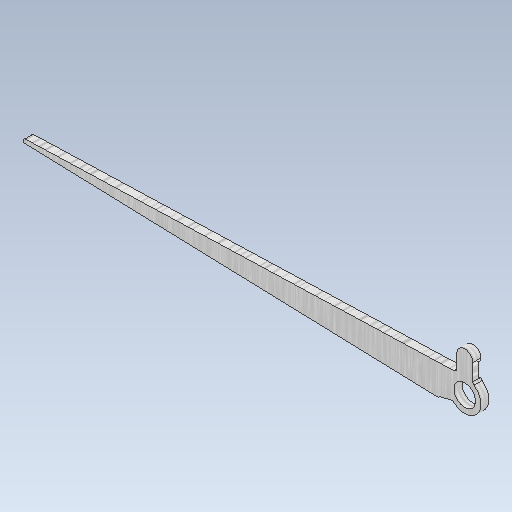
# Autodesk Inventor part: アーム先端
Saved by Autodesk Inventor 2020.2 (Build 242310000, 310)
## iProperties
Created: 2020-03-28
Part Number: アーム先端
Material: アルミニウム 7075
Document SubType Name: Modeling
Designer: aoyam
Density: 2.81 g/cm^3
Appearance: サテン - ブラシ仕上げ 重厚
Mass: 8.77948 g
Surface Area: 37.1512 cm^2
Volume: 3.12437 cm^3
Author: aoyam
Autodesk Inventor part; units mm, degrees
ref_plane "YZ Plane" through (0, 0, 0) normal (1, 0, 0) x (0, 1, 0)
ref_plane "XZ Plane" through (0, 0, 0) normal (0, 1, 0) x (-1, 0, 0)
ref_plane "XY Plane" through (0, 0, 0) normal (0, 0, 1) x (1, 0, 0)
sketch "スケッチ1" plane through (0, 0, 0) normal (0, 0, 1) x (1, 0, 0)
  line L0 (0, 0) -> (-164, 0)
  circle A0 centre (0, 0) radius 4.025
  line L1 (0, 0) -> (0, 12)
  circle A1 centre (0, 0) radius 6
  line L2 (0, 0) -> (0, 12) construction
  line L3 (3, 0) -> (3, 12)
  line L4 (-3, 12) -> (-3, 0)
  arc A2 (-3, 0) -> (3, 0) centre (0, 0) ccw
  arc A3 (3, 12) -> (-3, 12) centre (0, 12) ccw
  circle A4 centre (-164, 0) radius 0.75
  line L5 (-164.024, 0.7496) -> (-0.1921, 5.9969)
  line L6 (-0.1921, -5.9969) -> (-164.024, -0.7496)
  line L7 (-4.4505, -4.0241) -> (-11.6988, -5.6284)
  circle A5 centre (-7.8489, -7.8489) radius 3
  line L8 (0, 0) -> (-7.8489, -7.8489)
  line L9 (-139.5205, 0) -> (-135.0205, 7.7942)
  line L10 (-135.0205, 7.7942) -> (-164.1766, 0.7289)
  point P0 (0, 6)
  point P1 (3, 5.1962)
  point P2 (-3, 5.1962)
  point P3 (-8.4972, -4.9198)
  point P4 (-4.2426, -4.2426)
  point P5 (-9.9269, -5.6851)
  point P6 (-3, 5.907)
  point P7 (-138.6179, 1.5633)
  dimension "d2" = 164
  dimension "d3" = 8.05
  dimension "d4" = 12
  dimension "d5" = 90
  dimension "d7" = 6
  dimension "d8" = 1.5
  dimension "d13" = 6
  dimension "d14" = 45
  dimension "d21" = 12
  dimension "d23" = 11.1
  dimension "d33" = 30
  dimension "d34" = 9
  dimension "d35" = 60
  constraints: 24 end point, 10 point on circle, 10 tangent, 6 centre point, 2 coincident, 2 point on line, 1 horizontal, 1 midpoint, 1 parallel
  measures "d2" distance of L0.start L0.end
  measures "d3" diameter of A0
  measures "d4" distance of L1.start L1.end
  measures "d5" angle of L1 L0
  measures "d7" diameter of A3
  measures "d8" diameter of A4
  measures "d13" diameter of A5
  measures "d14" angle of L8 L0
  measures "d21" diameter of A1
  measures "d23" distance of L8.end L0.start
  measures "d33" distance of L9.end L10.end
  measures "d34" distance of L9.start L9.end
  measures "d35" angle of L0 L9
extrude "押し出し1" add sketch "スケッチ1" along normal blind 3 contours L1 A1 L3 A0 | A0 L4 A1 L1 | A0 L8 A1 L0 | L0 A1 L4 A0 | L3 A1 L8 A0 | A1 L5 L4 A3 L3 | A1 L7 L6 A4 L0 | L0 L9 L5 L4 A1 | L4 L5 A1 | L0 A4 L5 L9 | A4 | A5 L6 L7
fillet "フィレット1" radius 1.05 2 edges at (3, 5.1962, 1.5) (-9.9269, -5.6851, 1.5)
sketch "スケッチ2" plane through (0, 0, 3) normal (0, 0, 1) x (1, 0, 0)
  arc A0 (-10.3309, -5.6722) -> (-9.6625, -5.4591) centre (-10.2972, -4.6227) ccw projected
  arc A1 (-8.4972, -4.9198) -> (-9.6625, -5.4591) centre (-7.8489, -7.8489) ccw projected
  arc A2 (-4.4505, -4.0241) -> (3.4468, 4.9112) centre (0, 0) ccw projected
  arc A3 (3, 5.7706) -> (3.4468, 4.9112) centre (4.05, 5.7706) ccw projected
  line L0 (3, 5.7706) -> (3, 12) projected
  arc A4 (3, 12) -> (-3, 12) centre (0, 12) ccw projected
  line L1 (-3, 12) -> (-3, 5.907) projected
  line L2 (-3, 5.907) -> (-164.024, 0.7496) projected
  arc A5 (-164.024, 0.7496) -> (-164.024, -0.7496) centre (-164, 0) ccw projected
  line L3 (-164.024, -0.7496) -> (-10.3309, -5.6722) projected
  circle A6 centre (0, 0) radius 4.025 projected
  line L4 (-8.4972, -4.9198) -> (-4.4505, -4.0241) projected
fillet "フィレット3" radius 1.05 2 edges at (-4.4505, -4.0241, 1.5) (-3, 5.907, 1.5)
sketch "スケッチ4" plane through (0, 0, 0) normal (0, 0, -1) x (-1, 0, 0)
  circle A0 centre (0, 0) radius 4.025 projected
  arc A1 (9.6625, -5.4591) -> (10.3309, -5.6722) centre (10.2972, -4.6227) ccw projected
  line L0 (164.024, -0.7496) -> (10.3309, -5.6722) projected
  arc A2 (164.024, -0.7496) -> (164.024, 0.7496) centre (164, 0) ccw projected
  line L1 (4.0164, 5.8744) -> (164.024, 0.7496) projected
  arc A3 (3, 6.9239) -> (4.0164, 5.8744) centre (4.05, 6.9239) ccw projected
  line L2 (3, 12) -> (3, 6.9239) projected
  arc A4 (3, 12) -> (-3, 12) centre (0, 12) ccw projected
  line L3 (-3, 5.7706) -> (-3, 12) projected
  arc A5 (-3.4468, 4.9112) -> (-3, 5.7706) centre (-4.05, 5.7706) ccw projected
  arc A6 (-3.4468, 4.9112) -> (4.0752, -4.4037) centre (0, 0) ccw projected
  arc A7 (5.0153, -4.1491) -> (4.0752, -4.4037) centre (4.7884, -5.1743) ccw projected
  line L4 (8.4972, -4.9198) -> (5.0153, -4.1491) projected
  arc A8 (9.6625, -5.4591) -> (8.4972, -4.9198) centre (7.8489, -7.8489) ccw projected
  circle A9 centre (15.0911, 0) radius 2
  circle A10 centre (80.8845, 0) radius 1.05
  line L5 (15.12, 1.9998) -> (80.8997, 1.0499)
  line L6 (80.8997, -1.0499) -> (15.12, -1.9998)
  line L7 (0, 0) -> (80.8845, 0)
  dimension "d24" = 4
  dimension "d25" = 2.1
  constraints: 6 end point, 4 point on circle, 4 tangent, 2 centre point, 1 horizontal, 1 point on line
  measures "d24" diameter of A9
  measures "d25" diameter of A10
extrude "押し出し3" cut sketch "スケッチ4" against normal blind 1.5 contours L7 A9 | L7 A10 L6 A9 | A9 L7 | A9 L5 A10 L7 | A10
sketch "スケッチ5" plane through (0, 0, 0) normal (0, 0, -1) x (-1, 0, 0)
  line L0 (80.8997, -1.0499) -> (15.12, -1.9998) projected
  arc A0 (15.12, 1.9998) -> (15.12, -1.9998) centre (15.0911, 0) ccw projected
  line L1 (15.12, 1.9998) -> (80.8997, 1.0499) projected
  arc A1 (80.8997, -1.0499) -> (80.8997, 1.0499) centre (80.8845, 0) ccw projected
  circle A2 centre (0, 0) radius 4.025 projected
  arc A3 (9.6625, -5.4591) -> (10.3309, -5.6722) centre (10.2972, -4.6227) ccw projected
  line L2 (164.024, -0.7496) -> (10.3309, -5.6722) projected
  arc A4 (164.024, -0.7496) -> (164.024, 0.7496) centre (164, 0) ccw projected
  line L3 (4.0164, 5.8744) -> (164.024, 0.7496) projected
  arc A5 (3, 6.9239) -> (4.0164, 5.8744) centre (4.05, 6.9239) ccw projected
  line L4 (3, 12) -> (3, 6.9239) projected
  arc A6 (3, 12) -> (-3, 12) centre (0, 12) ccw projected
  line L5 (-3, 5.7706) -> (-3, 12) projected
  arc A7 (-3.4468, 4.9112) -> (-3, 5.7706) centre (-4.05, 5.7706) ccw projected
  arc A8 (-3.4468, 4.9112) -> (4.0752, -4.4037) centre (0, 0) ccw projected
  arc A9 (5.0153, -4.1491) -> (4.0752, -4.4037) centre (4.7884, -5.1743) ccw projected
  line L6 (8.4972, -4.9198) -> (5.0153, -4.1491) projected
  arc A10 (9.6625, -5.4591) -> (8.4972, -4.9198) centre (7.8489, -7.8489) ccw projected
  circle A11 centre (0, 8.5544) radius 2.55 construction
  circle A12 centre (0, 8.5544) radius 1.95
  line L7 (9.6625, 5.6936) -> (-9.679, 6.3131)
  line L8 (4.0164, 5.8744) -> (136.731, 1.6238) projected
  line L9 (0, 12) -> (0, 0)
  circle A13 centre (0, 8.5544) radius 4.05
  point P0 (-3.2264, 6.1064)
  point P1 (-3, 5.8336)
  point P2 (-3, 6.0992)
  point P3 (3.2928, 6.1965)
  point P4 (3.0632, 5.905)
  point P5 (-3, 11.2751)
  point P6 (3, 11.2751)
  point P7 (136.3385, 1.6363)
  dimension "d28" = 5.1
  dimension "d29" = 3.9
  dimension "d30" = 2.1
  constraints: 4 end point, 3 centre point, 2 point on line, 1 coincident, 1 collinear, 1 tangent
  measures "d28" diameter of A11
  measures "d29" diameter of A12
  measures "d30" radial gap between concentric circles of A12 A13
extrude "押し出し4" cut sketch "スケッチ5" against normal blind 1.05 contours L7 A13 A5 | A13 L7 L5 | L5 L7 L9 A13 | A13 L7 L5 L4 A5 | A5 L4 A13 | A13 L9 L7 | L7 A13 L5
